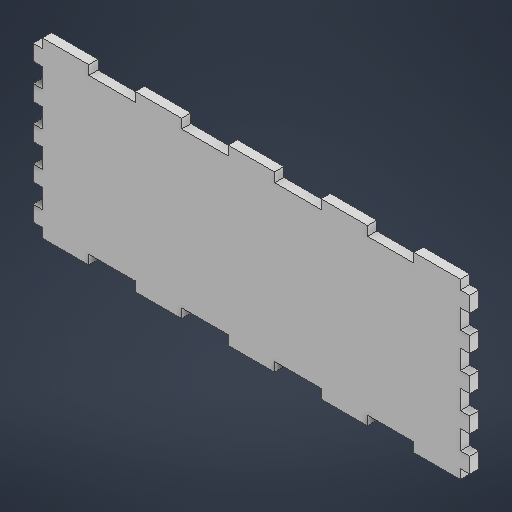
# Autodesk Inventor part: paredBase
Saved by Autodesk Inventor 2026 (Build 300175000, 175)
## iProperties
Created: 2026-04-21
Part Number: paredBase
Material: Generic
Document SubType Name: Modeling
Designer: juana
Density: 1 g/cm^3
Appearance: Default
Author: juana
Autodesk Inventor part; units mm, degrees
ref_plane "YZ Plane" through (0, 0, 0) normal (1, 0, 0) x (0, 1, 0)
ref_plane "XZ Plane" through (0, 0, 0) normal (0, 1, 0) x (-1, 0, 0)
ref_plane "XY Plane" through (0, 0, 0) normal (0, 0, 1) x (1, 0, 0)
sketch "Sketch1" plane through (0, 0, 0) normal (0, 0, 1) x (1, 0, 0)
  line L0 (0, 50) -> (135, 50)
  line L1 (135, 50) -> (135, 0)
  line L2 (135, 0) -> (0, 0)
  line L3 (0, 0) -> (0, 50)
  line L4 (-3, 50) -> (0, 50)
  line L5 (0, 50) -> (0, 45)
  line L6 (0, 45) -> (-3, 45)
  line L7 (-3, 45) -> (-3, 50)
  line L8 (-3, 38.75) -> (0, 38.75)
  line L9 (0, 38.75) -> (0, 33.75)
  line L10 (0, 33.75) -> (-3, 33.75)
  line L11 (-3, 33.75) -> (-3, 38.75)
  line L12 (-3, 27.5) -> (0, 27.5)
  line L13 (0, 27.5) -> (0, 22.5)
  line L14 (0, 22.5) -> (-3, 22.5)
  line L15 (-3, 22.5) -> (-3, 27.5)
  line L16 (135, 50) -> (138, 50)
  line L17 (138, 50) -> (138, 45)
  line L18 (138, 45) -> (135, 45)
  line L19 (135, 45) -> (135, 50)
  line L20 (135, 38.75) -> (138, 38.75)
  line L21 (138, 38.75) -> (138, 33.75)
  line L22 (138, 33.75) -> (135, 33.75)
  line L23 (135, 33.75) -> (135, 38.75)
  line L24 (135, 27.5) -> (138, 27.5)
  line L25 (138, 27.5) -> (138, 22.5)
  line L26 (138, 22.5) -> (135, 22.5)
  line L27 (135, 22.5) -> (135, 27.5)
  line L28 (0, 50) -> (15, 50)
  line L29 (15, 50) -> (15, 53)
  line L30 (15, 53) -> (0, 53)
  line L31 (0, 53) -> (0, 50)
  line L32 (30, 53) -> (30, 50)
  line L33 (30, 50) -> (45, 50)
  line L34 (45, 53) -> (30, 53)
  line L35 (45, 50) -> (45, 53)
  line L36 (60, 53) -> (60, 50)
  line L37 (60, 50) -> (75, 50)
  line L38 (75, 53) -> (60, 53)
  line L39 (75, 50) -> (75, 53)
  line L40 (90, 53) -> (90, 50)
  line L41 (90, 50) -> (105, 50)
  line L42 (105, 53) -> (90, 53)
  line L43 (105, 50) -> (105, 53)
  line L44 (120, 53) -> (120, 50)
  line L45 (120, 50) -> (135, 50)
  line L46 (135, 53) -> (120, 53)
  line L47 (135, 50) -> (135, 53)
  line L48 (0, 0) -> (0, -3)
  line L49 (0, -3) -> (15, -3)
  line L50 (15, 0) -> (0, 0)
  line L51 (15, -3) -> (15, 0)
  line L52 (30, 0) -> (30, -3)
  line L53 (30, -3) -> (45, -3)
  line L54 (45, 0) -> (30, 0)
  line L55 (45, -3) -> (45, 0)
  line L56 (60, 0) -> (60, -3)
  line L57 (60, -3) -> (75, -3)
  line L58 (75, 0) -> (60, 0)
  line L59 (75, -3) -> (75, 0)
  line L60 (90, 0) -> (90, -3)
  line L61 (90, -3) -> (105, -3)
  line L62 (105, 0) -> (90, 0)
  line L63 (105, -3) -> (105, 0)
  line L64 (120, 0) -> (120, -3)
  line L65 (120, -3) -> (135, -3)
  line L66 (135, 0) -> (120, 0)
  line L67 (135, -3) -> (135, 0)
  line L68 (-3, 16.25) -> (0, 16.25)
  line L69 (0, 16.25) -> (0, 11.25)
  line L70 (0, 11.25) -> (-3, 11.25)
  line L71 (-3, 11.25) -> (-3, 16.25)
  line L72 (135, 16.25) -> (138, 16.25)
  line L73 (138, 16.25) -> (138, 11.25)
  line L74 (138, 11.25) -> (135, 11.25)
  line L75 (135, 11.25) -> (135, 16.25)
  line L76 (-3, 5) -> (0, 5)
  line L77 (0, 5) -> (0, 0)
  line L78 (0, 0) -> (-3, 0)
  line L79 (-3, 0) -> (-3, 5)
  line L80 (135, 5) -> (138, 5)
  line L81 (138, 5) -> (138, 0)
  line L82 (138, 0) -> (135, 0)
  line L83 (135, 0) -> (135, 5)
  point P0 (15, 0)
  point P1 (30, 0)
  point P2 (45, 0)
  point P3 (60, 0)
  point P4 (90, 0)
  point P5 (105, 0)
  point P6 (120, 0)
  point P7 (135, 15)
  point P8 (0, 45)
  point P9 (0, 33.75)
  point P10 (0, 15)
  point P11 (135, 7)
  point P12 (0, 22.5)
  point P13 (0, 0)
  point P14 (0, 7)
  point P15 (135, 16.25)
  point P16 (135, 11.25)
  point P17 (135, 0)
  point P18 (0, 11.25)
  point P19 (135, 0)
  dimension "d0" = 50
  dimension "d1" = 135
  dimension "d2" = 3
  dimension "d3" = 5
  dimension "d6" = 11.25
  dimension "d9" = 138
  dimension "d12" = 3
  dimension "d13" = 15
  dimension "d16" = 30
  dimension "d19" = 53
  constraints: 168 end point, 6 parallel, 5 horizontal, 3 perpendicular, 2 vertical, 2 vertical alignment, 1 coincident, 1 horizontal alignment, 162 other
  measures "d0" distance of L0.end L1.end
  measures "d1" distance of L0.start L0.end
  measures "d2" distance of L4.start L4.end
  measures "d3" distance of L6.end L4.start
  measures "d6" distance of L0.start point (0, 38.75)
  measures "d9" distance of L0.start point (138, 50)
  measures "d12" distance of L30.end L4.end
  measures "d13" distance of L29.end L30.end
  measures "d16" distance of L0.start point (30, 50)
  measures "d19" distance of L0.start point (0, -3)
extrude "Extrusion1" add sketch "Sketch1" along normal blind 3
body "Solid1"
